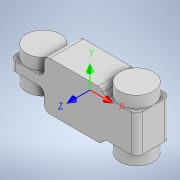
# Autodesk Inventor part: body
Saved by Autodesk Inventor 2020.2 (Build 242310000, 310)
## iProperties
Created: 2021-01-29
Part Number: body
Material: Generic
Document SubType Name: Modeling
Designer: DELL
Density: 1 g/cm^3
Appearance: Default
Author: DELL
Autodesk Inventor part; units mm, degrees
ref_plane "YZ Plane" through (0, 0, 0) normal (1, 0, 0) x (0, 1, 0)
ref_plane "XZ Plane" through (0, 0, 0) normal (0, 1, 0) x (-1, 0, 0)
ref_plane "XY Plane" through (0, 0, 0) normal (0, 0, 1) x (1, 0, 0)
sketch "Sketch1" plane through (0, 0, 0) normal (0, 0, 1) x (1, 0, 0)
  line L0 (-170, 13) -> (-77.5, 13)
  line L1 (170, 45) -> (170, 35)
  line L2 (-170, 0) -> (-170, 13)
  line L3 (-77.5, 65) -> (77.5, 65)
  line L4 (170, 50) -> (77.5, 50)
  line L5 (170, 0) -> (170, 50)
  line L6 (-77.5, 13) -> (-77.5, 65)
  line L7 (-170, 0) -> (170, 0) construction
  line L8 (77.5, 65) -> (77.5, 50)
  line L9 (62.5, 35) -> (155, 35)
  line L10 (155, 35) -> (155, 0)
  line L11 (-62.5, 0) -> (-62.5, 50)
  line L12 (-62.5, 50) -> (62.5, 50)
  line L13 (62.5, 50) -> (62.5, 35)
  line L14 (0, 50) -> (0, -50) construction
  line L15 (-238, 0) -> (238, 0) projected
  line L16 (0, -73) -> (0, 88) construction
  point P0 (0, 0)
  point P1 (170, 5)
  dimension "d15" = 0
  dimension "d2" = 155
  dimension "d21" = 92.5
  dimension "d25" = 92.5
  dimension "d29" = 15
  dimension "d30" = 26
  dimension "d31" = 15
  dimension "d32" = 15
  dimension "d33" = 100
  dimension "d34" = 15
  dimension "d35" = 100
  constraints: 30 end point, 5 point on line, 4 horizontal, 3 midpoint, 1 collinear, 1 parallel, 1 perpendicular, 1 vertical, 1 other
  measures "d2" distance of L3.start L3.end
  measures "d21" distance of L4.start L4.end
  measures "d25" distance between parallel lines of L6 L2
  measures "d29" distance between parallel lines of L4 L9
  measures "d30" diameter of L0 L15
  measures "d31" distance between parallel lines of L6 L11
  measures "d32" distance between parallel lines of L5 L10
  measures "d33" diameter of L4 L15
  measures "d34" distance between parallel lines of L8 L13
  measures "d35" diameter of L12 L15
extrude "Extrusion1" add sketch "Sketch1" along normal mid plane 90
sketch "Sketch2" plane through (0, 0, 0) normal (0, 1, 0) x (-1, 0, 0)
  circle A0 centre (-125, 0) radius 45
  circle A1 centre (125, 0) radius 45
  line L0 (238, 0) -> (-238, 0) projected
  line L1 (0, -63) -> (0, 63) projected
  point P0 (0, 0)
  dimension "d7" = 90
  dimension "d36" = 250
  constraints: 2 centre point, 1 equal radius, 1 point on line, 1 other
  measures "d7" diameter of A0
  measures "d36" diameter of A1.centre L1
extrude "Extrusion2" add sketch "Sketch2" along normal blind 32 from surface at 50 contours L0 A0 | A0 L0
extrude "Extrusion3" add sketch "Sketch2" along normal blind 32 from surface at 13 contours L0 A1 | A1 L0
extrude "Extrusion4" cut sketch "Sketch1" against normal mid plane 55 contours L11 L12 L13 L9 L10 L15
fillet "Fillet1" radius 15 12 edges at (77.5, 65, 0) (-77.5, 65, 0) (-62.5, 50, 0) (155, 35, 0) (-170, 6.5, 45) (-170, 6.5, -45) (170, 25, -45) (170, 25, 45) (62.5, 50, 0) (62.5, 35, 0) (77.5, 50, 0) (-77.5, 13, 0)
mirror "Mirror1" about plane through (0, 0, 0) normal (0, 1, 0)
body "Solid1"
